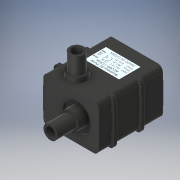
# Autodesk Inventor part: AD20P-1230A DC Pump
Saved by Autodesk Inventor 2019 (Build 230136000, 136)
## iProperties
Created: 2019-12-27
Part Number: AD20P-1230A DC Pump
Material: Generic
Document SubType Name: Modeling
Designer: anggitoz
Mass: 37.2319 g
Surface Area: 89.8677 cm^2
Volume: 37.2319 cm^3
Density: 1 g/cm^3
Appearance: Smooth - Black
Author: anggitoz
Autodesk Inventor part; units mm, degrees
ref_plane "YZ Plane" through (0, 0, 0) normal (1, 0, 0) x (0, 1, 0)
ref_plane "XZ Plane" through (0, 0, 0) normal (0, 1, 0) x (-1, 0, 0)
sketch "Sketch1" plane through (0, 0, 0) normal (0, 0, 1) x (1, 0, 0)
  line L0 (2.8104, 0) -> (30.1896, 0)
  line L1 (33, 0) -> (33, 27.5) construction
  line L2 (30.1896, 27.5) -> (2.8104, 27.5)
  line L3 (0, 27.5) -> (0, 0) construction
  line L4 (-0.5, 13.75) -> (33.5, 13.75) construction
  arc A0 (-0.1846, 24.6731) -> (-0.1846, 2.8269) centre (188.8125, 13.75) ccw
  arc A1 (33.1846, 2.8269) -> (33.1846, 24.6731) centre (-155.8125, 13.75) ccw
  arc A2 (2.8104, 27.5) -> (-0.1846, 24.6731) centre (2.8104, 24.5) ccw
  arc A3 (33.1846, 24.6731) -> (30.1896, 27.5) centre (30.1896, 24.5) ccw
  arc A4 (-0.1846, 2.8269) -> (2.8104, 0) centre (2.8104, 3) ccw
  arc A5 (30.1896, 0) -> (33.1846, 2.8269) centre (30.1896, 3) ccw
  dimension "d0" = 33
  dimension "d1" = 27.5
  dimension "d2" = 0.5
  dimension "d3" = 0.5
  dimension "d4" = 3
  constraints: 18 point on circle, 10 end point, 8 tangent, 6 centre point, 4 point on line, 3 equal radius, 2 horizontal, 2 parallel, 1 perpendicular
  measures "d0" distance of L3.start L1.end
  measures "d1" distance of L1.end L1.start
  measures "d2" distance from line of L3 L4.start
  measures "d3" distance from line of L1 L4.end
  measures "d4" radius of A2
extrude "Extrusion1" add sketch "Sketch1" along normal mid plane 39
ref_plane "Work Plane1" through (0, 0, 2.5) normal (0, 0, 1) x (1, 0, 0)
sketch "Sketch2" plane through (0, 0, 2.5) normal (0, 0, 1) x (1, 0, 0)
  arc A0 (2.8104, 27.5) -> (-0.1846, 24.6731) centre (2.8104, 24.5) ccw projected
  arc A1 (-0.1846, 24.6731) -> (-0.1846, 2.8269) centre (188.8125, 13.75) ccw projected
  arc A2 (-0.1846, 2.8269) -> (2.8104, 0) centre (2.8104, 3) ccw projected
  line L0 (2.8104, 0) -> (30.1896, 0) projected
  arc A3 (30.1896, 0) -> (33.1846, 2.8269) centre (30.1896, 3) ccw projected
  arc A4 (33.1846, 2.8269) -> (33.1846, 24.6731) centre (-155.8125, 13.75) ccw projected
  arc A5 (33.1846, 24.6731) -> (30.1896, 27.5) centre (30.1896, 24.5) ccw projected
  line L1 (30.1896, 27.5) -> (2.8104, 27.5) projected
  arc A6 (-0.1846, 24.6731) -> (-0.1846, 2.8269) centre (188.8125, 13.75) ccw projected
  line L2 (-0.5, 13.75) -> (33.5, 13.75) construction
  arc A7 (-1.3139, 26.3) -> (-1.6821, 24.7596) centre (2.8104, 24.5) ccw
  arc A8 (34.6821, 24.7596) -> (34.3139, 26.3) centre (30.1896, 24.5) ccw
  arc A9 (34.6821, 2.7404) -> (34.6821, 24.7596) centre (-155.8125, 13.75) ccw
  arc A10 (34.3139, 1.2) -> (34.6821, 2.7404) centre (30.1896, 3) ccw
  arc A11 (-1.6821, 2.7404) -> (-1.3139, 1.2) centre (2.8104, 3) ccw
  line L3 (0.5191, 27.5) -> (32.4809, 27.5)
  line L4 (0.5191, 0) -> (32.4809, 0)
  arc A12 (-1.6821, 24.7596) -> (-1.6821, 2.7404) centre (188.8125, 13.75) ccw
  arc A13 (34.3139, 26.3) -> (32.4809, 27.5) centre (32.4809, 25.5) ccw
  arc A14 (0.5191, 27.5) -> (-1.3139, 26.3) centre (0.5191, 25.5) ccw
  arc A15 (-1.3139, 1.2) -> (0.5191, 0) centre (0.5191, 2) ccw
  arc A16 (32.4809, 0) -> (34.3139, 1.2) centre (32.4809, 2) ccw
  point P0 (0, 0)
  point P1 (33.5437, 27.5)
  point P2 (33.5437, 0)
  point P3 (-0.5437, 0)
  point P4 (-0.5437, 27.5)
  dimension "d9" = 1.5
  dimension "d10" = 2
  dimension "d11" = 2
  dimension "d12" = 2
  dimension "d13" = 2
  constraints: 27 point on circle, 10 centre point, 8 tangent, 6 end point, 4 point on line, 2 horizontal
  measures "d9" radial gap between concentric circles of A1 A12
  measures "d10" radius of A13
  measures "d11" radius of A14
  measures "d12" radius of A15
  measures "d13" radius of A16
extrude "Extrusion2" add sketch "Sketch2" along normal mid plane 18.5 contours A0 A1 A2 L4 A15 A11 A12 A7 A14 L3 | L3 A13 A8 A9 A10 A16 L4 A3 A4 A5
sketch "Sketch3" plane through (0, 0, 2.5) normal (0, 0, 1) x (1, 0, 0)
  arc A0 (-0.1846, 2.8269) -> (2.8104, 0) centre (2.8104, 3) ccw projected
  arc A1 (-0.1846, 24.6731) -> (-0.1846, 2.8269) centre (188.8125, 13.75) ccw projected
  arc A2 (2.8104, 27.5) -> (-0.1846, 24.6731) centre (2.8104, 24.5) ccw projected
  line L0 (2.8104, 27.5) -> (0.5191, 27.5) projected
  arc A3 (0.5191, 27.5) -> (-1.3139, 26.3) centre (0.5191, 25.5) ccw projected
  arc A4 (-1.3139, 26.3) -> (-1.6821, 24.7596) centre (2.8104, 24.5) ccw projected
  arc A5 (-1.6821, 24.7596) -> (-1.6821, 2.7404) centre (188.8125, 13.75) ccw projected
  arc A6 (-1.6821, 2.7404) -> (-1.3139, 1.2) centre (2.8104, 3) ccw projected
  arc A7 (-1.3139, 1.2) -> (0.5191, 0) centre (0.5191, 2) ccw projected
  line L1 (0.5191, 0) -> (2.8104, 0) projected
  arc A8 (30.1896, 0) -> (33.1846, 2.8269) centre (30.1896, 3) ccw projected
  line L2 (30.1896, 0) -> (32.4809, 0) projected
  arc A9 (32.4809, 0) -> (34.3139, 1.2) centre (32.4809, 2) ccw projected
  arc A10 (34.3139, 1.2) -> (34.6821, 2.7404) centre (30.1896, 3) ccw projected
  arc A11 (34.6821, 2.7404) -> (34.6821, 24.7596) centre (-155.8125, 13.75) ccw projected
  arc A12 (34.6821, 24.7596) -> (34.3139, 26.3) centre (30.1896, 24.5) ccw projected
  arc A13 (34.3139, 26.3) -> (32.4809, 27.5) centre (32.4809, 25.5) ccw projected
  line L3 (32.4809, 27.5) -> (30.1896, 27.5) projected
  arc A14 (33.1846, 24.6731) -> (30.1896, 27.5) centre (30.1896, 24.5) ccw projected
  arc A15 (33.1846, 2.8269) -> (33.1846, 24.6731) centre (-155.8125, 13.75) ccw projected
  point P0 (0, 0)
extrude "Extrusion3" cut sketch "Sketch3" along normal mid plane 14.7
sketch "Sketch4" plane through (2.8104, 0, -19.5) normal (0, -1, 0) x (1, 0, 0)
  line L0 (27.3792, 39) -> (0, 39) construction
  line L1 (13.6896, 39) -> (13.6896, 22) construction
  line L2 (13.6896, 22) -> (-8.8104, 22) construction
  line L3 (13.6896, 22) -> (36.1896, 22) construction
  line L4 (9.3896, 51.4625) -> (9.3896, -5.4859) construction
  line L5 (17.1896, 54.9508) -> (17.1896, -9.4609) construction
  line L6 (-8.8104, 31.25) -> (38.6008, 31.25) construction
  point P0 (-2.8104, 19.5)
  dimension "d18" = 17
  dimension "d19" = 22.5
  dimension "d20" = 22.5
  dimension "d21" = 26.8
  dimension "d22" = 7.8
  constraints: 12 end point, 3 vertical, 1 horizontal, 1 midpoint, 1 perpendicular, 1 point on line
  measures "d18" distance of L1.start L1.end
  measures "d19" distance of L1.end L2.end
  measures "d20" distance of L1.end L3.end
  measures "d21" distance from line of L3.end L4
  measures "d22" distance between parallel lines of L5 L4
sketch "Sketch5" plane through (2.8104, 27.5, 19.5) normal (0, 1, 0) x (1, 0, 0)
  line L0 (-8.8104, 7.75) -> (38.6008, 7.75) construction
  line L1 (13.6896, 17) -> (36.1896, 17) construction
  line L2 (17.1896, -15.9508) -> (17.1896, 48.4609) construction
  line L3 (9.3896, -12.4625) -> (9.3896, 44.4859) construction
  line L4 (13.6896, 17) -> (-8.8104, 17) construction
  circle A0 centre (9.3896, 7.75) radius 5.5
  circle A1 centre (9.3896, 7.75) radius 4.25
  point P0 (-2.8104, 19.5)
  dimension "d23" = 11
  dimension "d24" = 8.5
  constraints: 2 centre point, 2 point on line, 1 coincident
  measures "d23" diameter of A0
  measures "d24" diameter of A1
extrude "Extrusion4" add sketch "Sketch5" along normal blind 3
sketch "Sketch6" plane through (2.8104, 27.5, 19.5) normal (0, 1, 0) x (1, 0, 0)
  circle A0 centre (9.3896, 7.75) radius 4.25 projected
  point P0 (-2.8104, 19.5)
extrude "Extrusion5" add sketch "Sketch6" along normal blind 13.4
sketch "Sketch7" plane through (12.2, 40.9, 11.75) normal (0, 1, 0) x (1, 0, 0)
  point P0 (-12.2, 11.75)
  point P1 (-0.0229, 0.0053)
hole "Hole1" at (12.1771, 40.9, 11.7447) direction (0, -1, 0) diameter 6 depth 13.4 tip angle 118
sketch "Sketch8" plane through (0, 0, 19.5) normal (0, 0, 1) x (1, 0, 0)
  line L0 (16.45, 40.9) -> (7.95, 40.9) construction
  line L1 (7.95, 30.5) -> (16.45, 30.5) construction
  arc A0 (2.8104, 27.5) -> (-0.1846, 24.6731) centre (2.8104, 24.5) ccw construction
  arc A1 (-0.1846, 24.6731) -> (-0.1846, 2.8269) centre (188.8125, 13.75) ccw construction
  arc A2 (-0.1846, 2.8269) -> (2.8104, 0) centre (2.8104, 3) ccw construction
  line L2 (2.8104, 0) -> (30.1896, 0) construction
  arc A3 (30.1896, 0) -> (33.1846, 2.8269) centre (30.1896, 3) ccw construction
  arc A4 (33.1846, 2.8269) -> (33.1846, 24.6731) centre (-155.8125, 13.75) ccw construction
  arc A5 (33.1846, 24.6731) -> (30.1896, 27.5) centre (30.1896, 24.5) ccw construction
  line L3 (30.1896, 27.5) -> (2.8104, 27.5) construction
  line L4 (-10.3414, 13.75) -> (38.9041, 13.75) construction
  circle A6 centre (20, 13.75) radius 5.5
  line L5 (12.2, 42.7052) -> (12.2, 21.084) construction
  point P0 (0, 0)
  dimension "d36" = 11
  dimension "d37" = 7.8
  constraints: 4 end point, 1 centre point, 1 horizontal, 1 point on line, 1 vertical
  measures "d36" diameter of A6
  measures "d37" distance from line of A6.centre L5
extrude "Extrusion6" add sketch "Sketch8" along normal blind 4.5
sketch "Sketch9" plane through (20, 13.75, 24) normal (0, 0, 1) x (1, 0, 0)
  circle A0 centre (0, 0) radius 4.2
  point P0 (-20, -13.75)
  dimension "d40" = 8.4
  constraints: 1 centre point
  measures "d40" diameter of A0
extrude "Extrusion7" add sketch "Sketch9" along normal blind 11.5
sketch "Sketch10" plane through (20, 13.75, 35.5) normal (0, 0, 1) x (1, 0, 0)
  point P0 (-20, -13.75)
  point P1 (0, 0)
hole "Hole2" at (20, 13.75, 35.5) direction (0, 0, -1) diameter 6 depth 13.4 tip angle 118
sketch "Sketch11" plane through (0, 0, 19.5) normal (0, 0, 1) x (1, 0, 0)
  circle A0 centre (20, 13.75) radius 5.5 projected
  arc A1 (2.8104, 27.5) -> (-0.1846, 24.6731) centre (2.8104, 24.5) ccw projected
  arc A2 (-0.1846, 24.6731) -> (-0.1846, 2.8269) centre (188.8125, 13.75) ccw projected
  arc A3 (-0.1846, 2.8269) -> (2.8104, 0) centre (2.8104, 3) ccw projected
  line L0 (2.8104, 0) -> (30.1896, 0) projected
  arc A4 (30.1896, 0) -> (33.1846, 2.8269) centre (30.1896, 3) ccw projected
  arc A5 (33.1846, 2.8269) -> (33.1846, 24.6731) centre (-155.8125, 13.75) ccw projected
  arc A6 (33.1846, 24.6731) -> (30.1896, 27.5) centre (30.1896, 24.5) ccw projected
  line L1 (30.1896, 27.5) -> (2.8104, 27.5) projected
  arc A7 (2.8104, 26.5) -> (0.8137, 24.6154) centre (2.8104, 24.5) ccw
  arc A8 (0.8137, 24.6154) -> (0.8137, 2.8846) centre (188.8125, 13.75) ccw
  arc A9 (0.8137, 2.8846) -> (2.8104, 1) centre (2.8104, 3) ccw
  line L2 (2.8104, 1) -> (30.1896, 1)
  arc A10 (30.1896, 1) -> (32.1863, 2.8846) centre (30.1896, 3) ccw
  arc A11 (32.1863, 2.8846) -> (32.1863, 24.6154) centre (-155.8125, 13.75) ccw
  arc A12 (32.1863, 24.6154) -> (30.1896, 26.5) centre (30.1896, 24.5) ccw
  line L3 (30.1896, 26.5) -> (2.8104, 26.5)
  arc A13 (2.8104, 26.3) -> (1.0134, 24.6039) centre (2.8104, 24.5) ccw
  line L4 (2.8104, 26.3) -> (30.1896, 26.3)
  arc A14 (31.9866, 24.6039) -> (30.1896, 26.3) centre (30.1896, 24.5) ccw
  arc A15 (31.9866, 2.8961) -> (31.9866, 24.6039) centre (-155.8125, 13.75) ccw
  arc A16 (30.1896, 1.2) -> (31.9866, 2.8961) centre (30.1896, 3) ccw
  line L5 (30.1896, 1.2) -> (2.8104, 1.2)
  arc A17 (1.0134, 2.8961) -> (2.8104, 1.2) centre (2.8104, 3) ccw
  arc A18 (1.0134, 24.6039) -> (1.0134, 2.8961) centre (188.8125, 13.75) ccw
  line L6 (-3.7926, 13.75) -> (36.6452, 13.75) construction
  point P0 (0, 0)
  dimension "d50" = 1
  dimension "d51" = 0.2
  constraints: 24 point on circle, 12 centre point, 10 end point, 1 horizontal, 14 other
  measures "d50" distance between parallel lines of L1 L3
  measures "d51" radial gap between concentric circles of A7 A13
extrude "Extrusion8" cut sketch "Sketch11" against normal blind 2 contours L3 A12 A11 A10 L2 A9 A8 A7
sketch "Sketch12" plane through (0, 0, -19.5) normal (0, 0, -1) x (-1, 0, 0)
  arc A0 (-1.0134, 2.8961) -> (-1.0134, 24.6039) centre (-188.8125, 13.75) ccw projected
  arc A1 (-2.8104, 1.2) -> (-1.0134, 2.8961) centre (-2.8104, 3) ccw projected
  line L0 (-2.8104, 1.2) -> (-30.1896, 1.2) projected
  arc A2 (-31.9866, 2.8961) -> (-30.1896, 1.2) centre (-30.1896, 3) ccw projected
  arc A3 (-31.9866, 24.6039) -> (-31.9866, 2.8961) centre (155.8125, 13.75) ccw projected
  arc A4 (-30.1896, 26.3) -> (-31.9866, 24.6039) centre (-30.1896, 24.5) ccw projected
  line L1 (-30.1896, 26.3) -> (-2.8104, 26.3) projected
  arc A5 (-1.0134, 24.6039) -> (-2.8104, 26.3) centre (-2.8104, 24.5) ccw projected
  circle A6 centre (-20, 13.75) radius 5.5 projected
  arc A7 (0.1846, 24.6731) -> (-2.8104, 27.5) centre (-2.8104, 24.5) ccw projected
  arc A8 (0.1846, 2.8269) -> (0.1846, 24.6731) centre (-188.8125, 13.75) ccw projected
  arc A9 (-2.8104, 0) -> (0.1846, 2.8269) centre (-2.8104, 3) ccw projected
  line L2 (-2.8104, 0) -> (-30.1896, 0) projected
  arc A10 (-33.1846, 2.8269) -> (-30.1896, 0) centre (-30.1896, 3) ccw projected
  arc A11 (-33.1846, 24.6731) -> (-33.1846, 2.8269) centre (155.8125, 13.75) ccw projected
  arc A12 (-30.1896, 27.5) -> (-33.1846, 24.6731) centre (-30.1896, 24.5) ccw projected
  line L3 (-30.1896, 27.5) -> (-2.8104, 27.5) projected
  arc A13 (-0.8137, 2.8846) -> (-0.8137, 24.6154) centre (-188.8125, 13.75) ccw projected
  arc A14 (-0.8137, 24.6154) -> (-2.8104, 26.5) centre (-2.8104, 24.5) ccw projected
  line L4 (-2.8104, 26.5) -> (-30.1896, 26.5) projected
  arc A15 (-30.1896, 26.5) -> (-32.1863, 24.6154) centre (-30.1896, 24.5) ccw projected
  arc A16 (-32.1863, 24.6154) -> (-32.1863, 2.8846) centre (155.8125, 13.75) ccw projected
  arc A17 (-32.1863, 2.8846) -> (-30.1896, 1) centre (-30.1896, 3) ccw projected
  line L5 (-30.1896, 1) -> (-2.8104, 1) projected
  arc A18 (-2.8104, 1) -> (-0.8137, 2.8846) centre (-2.8104, 3) ccw projected
  point P0 (0, 0)
extrude "Extrusion9" cut sketch "Sketch12" against normal blind 2 contours A18 L5 A17 A16 A15 L4 A14 A13
sketch "Sketch13" plane through (2.8104, 27.5, 19.5) normal (0, 1, 0) x (1, 0, 0)
  line L0 (23.9941, 18.8458) -> (2.9639, 18.8458) construction
  line L1 (2.9639, 18.8458) -> (2.9639, 31.9339) construction
  line L2 (2.9639, 31.9339) -> (23.9941, 31.9339) construction
  line L3 (23.9941, 31.9339) -> (23.9941, 18.8458) construction
  point P0 (-2.8104, 19.5)
  constraints: 2 other
decal "Decal1"
sketch "Sketch14" plane through (0, 0, 19.5) normal (0, 0, 1) x (1, 0, 0)
  arc A0 (1.0134, 24.6039) -> (1.0134, 2.8961) centre (188.8125, 13.75) ccw projected
  arc A1 (1.0134, 2.8961) -> (2.8104, 1.2) centre (2.8104, 3) ccw projected
  line L0 (2.8104, 1.2) -> (30.1896, 1.2) projected
  arc A2 (30.1896, 1.2) -> (31.9866, 2.8961) centre (30.1896, 3) ccw projected
  arc A3 (31.9866, 2.8961) -> (31.9866, 24.6039) centre (-155.8125, 13.75) ccw projected
  arc A4 (31.9866, 24.6039) -> (30.1896, 26.3) centre (30.1896, 24.5) ccw projected
  line L1 (30.1896, 26.3) -> (2.8104, 26.3) projected
  arc A5 (2.8104, 26.3) -> (1.0134, 24.6039) centre (2.8104, 24.5) ccw projected
  circle A6 centre (20, 13.75) radius 5.5 projected
  circle A7 centre (20, 13.75) radius 8.5
  point P0 (0, 0)
  dimension "d81" = 17
  constraints: 1 centre point, 1 coincident
  measures "d81" diameter of A7
extrude "Extrusion10" cut sketch "Sketch14" against normal blind 2 contours A7
body "Solid1"
